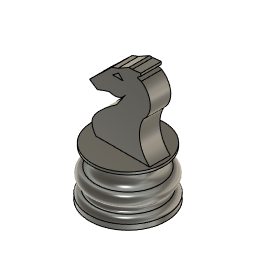
Knight v1 (Autodesk Fusion 360 design; units mm, degrees)
Autodesk Fusion 360 part; units mm, degrees
sketch "Sketch1" plane through (0, 0, 0) normal (0, 1, 0) x (1, 0, 0)
  line L0 (0, 0) -> (12.5, 0)
  line L1 (0, 0) -> (12.5, 0)
  line L2 (0, 0) -> (12.5, 0)
  line L3 (13, -1) -> (15, -1)
  line L4 (12.5, 0) -> (12.5, -1)
  line L5 (12.5, -1) -> (13, -1)
  line L6 (15, -1) -> (15, -3)
  arc A0 (13.0004, -5.0007) -> (15, -3) centre (12.9993, -3) ccw
  arc A1 (12.5, -12.1581) -> (12.5, -7.5136) centre (12.5473, -9.8359) ccw
  arc A2 (13.0004, -5.0007) -> (12.5, -7.5136) centre (13.0198, -6.3108) ccw
  arc A3 (12.5, -12.1581) -> (10.5425, -17.2326) centre (12.8282, -15.1996) ccw
  line L7 (0, 0) -> (0, -50)
  arc A4 (10.5425, -17.2326) -> (14, -19) centre (14, -14.7343) ccw
  line L8 (14, -19) -> (14, -20)
  line L9 (14, -20) -> (0, -20)
  dimension "d3" = 50
  constraint coincident L0.start L1.start
  constraint horizontal L0
  constraint parallel L0 L1
  constraint parallel L2 L3
  constraint perpendicular L2 L4
  constraint perpendicular L4 L5
  constraint perpendicular L3 L6
  constraint tangent L6 A0
  constraint perpendicular L1 L7
  constraint coincident L7 L9.end
  constraint perpendicular L7 L9
  measures "d3" distance of L0.start L7.end
revolve "Revolve1" add sketch "Sketch1" angle 360 about axis through (0, 0, 0) along (0, 0, 1)
sketch "Sketch2" plane through (0, 0, 0) normal (0, 1, 0) x (1, 0, 0)
  line L0 (2.9679, -49.4207) -> (3.0294, -49.543)
  line L1 (4.3602, -49.6653) -> (5.68, -49.6653)
  line L2 (5.68, -49.6653) -> (9, -50)
  line L3 (9, -50) -> (9, -49)
  line L4 (9, -49) -> (7.5814, -47.8487)
  arc A0 (9.1888, -47.3735) -> (10, -35) centre (4.9813, -40.8843) ccw
  arc A1 (12.5, -20) -> (10, -35) centre (20.625, -29.0625) ccw
  line L5 (0.0971, -47.2642) -> (4.3602, -49.6653)
  line L6 (0.0971, -47.2642) -> (-2.3608, -46.3487)
  arc A2 (0, -36.5) -> (-0.5465, -34.5722) centre (-1.7713, -35.9608) ccw
  arc A3 (-8.5, -20) -> (-10, -25) centre (-3.8456, -24.1213) ccw
  line L7 (-8.5, -20) -> (12.5, -20)
  spline S0 degree 5 poles (-0.5465, -34.5722) (-1.0465, -34.2231) (-2.0194, -33.5294) (-3.3975, -32.5026) (-5.0695, -31.1616) (-6.8628, -29.5355) (-8.3256, -27.9653) (-9.2046, -26.7511) (-9.6767, -25.8703) (-9.9047, -25.2953) (-9.9975, -25.0078) (-10, -25) knots 0 0 0 0 0 0 0.1 0.2 0.3 0.4 0.5 0.6 0.602776 0.602776 0.602776 0.602776 0.602776 0.602776
  line L8 (-9.7194, -25.875) -> (-10.2806, -24.125)
  line L9 (-2.3608, -46.3487) -> (-11, -38)
  line L10 (-11, -38) -> (-8, -36)
  line L11 (-8, -36) -> (-5.3151, -37)
  line L12 (-5.3151, -37) -> (-3.202, -37.6423)
  line L13 (2.8801, -39.491) -> (-0.242, -34.9169)
  line L14 (7.5814, -47.8487) -> (9.1888, -47.3735)
  arc A4 (2.8801, -39.491) -> (-3.202, -37.6423) centre (-1.3116, -42.3521) ccw
  line L15 (2, -44) -> (0.3442, -45.7134)
  line L16 (0.3442, -45.7134) -> (-2, -44)
  line L17 (-2, -44) -> (2, -44)
  constraint vertical L3
  constraint horizontal L7
  constraint midpoint A3.end L8
  constraint parallel L6 L11
  constraint coincident A2 L13.end
  constraint tangent A2 L13
  constraint tangent L13 A4
  constraint perpendicular L9 L15
  constraint horizontal L17
extrude "Extrude2" add sketch "Sketch2" along normal blind 4 and the other way blind 4
